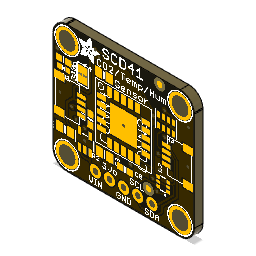
Board (Autodesk Fusion 360 design; units mm, degrees)
Autodesk Fusion 360 part; units mm, degrees
sketch "Outline" plane through (0, 0, 0) normal (0, 0, 1) x (1, 0, 0)
  arc A0 (0, 2.54) -> (2.54, 0) centre (2.54, 2.54) ccw
  arc A1 (23.0814, 0.0097) -> (25.4, 2.54) centre (22.86, 2.54) ccw
  arc A2 (25.3903, 20.5414) -> (22.86, 22.86) centre (22.86, 20.32) ccw
  arc A3 (2.3186, 22.8503) -> (0, 20.32) centre (2.54, 20.32) ccw
  line L0 (2.54, 0) -> (22.86, 0)
  line L1 (22.86, 0) -> (23.0814, 0.0097)
  line L2 (25.4, 2.54) -> (25.4, 20.32)
  line L3 (25.4, 20.32) -> (25.3903, 20.5414)
  line L4 (22.86, 22.86) -> (2.54, 22.86)
  line L5 (2.54, 22.86) -> (2.3186, 22.8503)
  line L6 (0, 20.32) -> (0, 2.54)
extrude "Extrude1" add sketch "Outline" along normal blind 1.57
named bodies: "Board"
